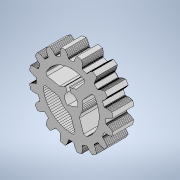
# Autodesk Inventor part: Ведущая шестерня дифференециала
Saved by Autodesk Inventor 2020 (Build 240168000, 168)
## iProperties
Created: 2021-05-23
Part Number: Ведущая шестерня дифференециала
Material: Типовые
Document SubType Name: Modeling
Designer: Антон
Density: 1 g/cm^3
Appearance: По умолчанию
Author: Антон
Autodesk Inventor part; units mm, degrees
note: some values were not read from the file. Chosen so that the rebuilt part matches the saved one: arc direction of "Выдавливание3".
(part 1 of 2)
ref_plane "YZ Plane" through (0, 0, 0) normal (1, 0, 0) x (0, 1, 0)
ref_plane "XZ Plane" through (0, 0, 0) normal (0, 1, 0) x (-1, 0, 0)
ref_plane "XY Plane" through (0, 0, 0) normal (0, 0, 1) x (1, 0, 0)
sketch "Эскиз1" plane through (0, 0, 0) normal (0, 0, 1) x (1, 0, 0)
  line L0 (0.5652, 9.3598) -> (0.528, 9.4555)
  line L1 (0.528, 9.4555) -> (0.4873, 9.4932)
  line L2 (0.4873, 9.4932) -> (0.446, 9.5204)
  line L3 (0.446, 9.5204) -> (0.3622, 9.5591)
  line L4 (0.3622, 9.5591) -> (0.2775, 9.5854)
  line L5 (0.2775, 9.5854) -> (0.1922, 9.604)
  line L6 (0.1922, 9.604) -> (0.0227, 9.6523)
  line L7 (0.0227, 9.6523) -> (-0.1453, 9.7165)
  line L8 (-0.1453, 9.7165) -> (-0.3118, 9.7933)
  line L9 (-0.3118, 9.7933) -> (-0.4767, 9.881)
  line L10 (-0.4767, 9.881) -> (-0.6399, 9.9788)
  line L11 (-0.6399, 9.9788) -> (-0.8013, 10.0859)
  line L12 (-0.8013, 10.0859) -> (-0.9608, 10.202)
  line L13 (-0.9608, 10.202) -> (-1.0789, 10.2947)
  line L14 (-1.0789, 10.2947) -> (-0.8657, 11.3669)
  line L15 (-0.8657, 11.3669) -> (-0.721, 11.4073)
  line L16 (-0.721, 11.4073) -> (-0.5293, 11.4535)
  line L17 (-0.5293, 11.4535) -> (-0.3392, 11.4907)
  line L18 (-0.3392, 11.4907) -> (-0.151, 11.5186)
  line L19 (-0.151, 11.5186) -> (0.035, 11.5365)
  line L20 (0.035, 11.5365) -> (0.2181, 11.5437)
  line L21 (0.2181, 11.5437) -> (0.3979, 11.5388)
  line L22 (0.3979, 11.5388) -> (0.573, 11.5185)
  line L23 (0.573, 11.5185) -> (0.659, 11.5031)
  line L24 (0.659, 11.5031) -> (0.7473, 11.4949)
  line L25 (0.7473, 11.4949) -> (0.8395, 11.4986)
  line L26 (0.8395, 11.4986) -> (0.8881, 11.5079)
  line L27 (0.8881, 11.5079) -> (0.9401, 11.5272)
  line L28 (0.9401, 11.5272) -> (1.0111, 11.6014)
  line L29 (1.0111, 11.6014) -> (1.3841, 12.5018)
  line L30 (1.3841, 12.5018) -> (1.3863, 12.6044)
  line L31 (1.3863, 12.6044) -> (1.3631, 12.6548)
  line L32 (1.3631, 12.6548) -> (1.3354, 12.6958)
  line L33 (1.3354, 12.6958) -> (1.2728, 12.7636)
  line L34 (1.2728, 12.7636) -> (1.2046, 12.8203)
  line L35 (1.2046, 12.8203) -> (1.1329, 12.8702)
  line L36 (1.1329, 12.8702) -> (0.9947, 12.9796)
  line L37 (0.9947, 12.9796) -> (0.8641, 13.1032)
  line L38 (0.8641, 13.1032) -> (0.7397, 13.2378)
  line L39 (0.7397, 13.2378) -> (0.6209, 13.382)
  line L40 (0.6209, 13.382) -> (0.5075, 13.5348)
  line L41 (0.5075, 13.5348) -> (0.3994, 13.6956)
  line L42 (0.3994, 13.6956) -> (0.2965, 13.8638)
  line L43 (0.2965, 13.8638) -> (0.2228, 13.9947)
  line L44 (0.2228, 13.9947) -> (0.8302, 14.9036)
  line L45 (0.8302, 14.9036) -> (0.9793, 14.8856)
  line L46 (0.9793, 14.8856) -> (1.1741, 14.8549)
  line L47 (1.1741, 14.8549) -> (1.364, 14.8166)
  line L48 (1.364, 14.8166) -> (1.5485, 14.7703)
  line L49 (1.5485, 14.7703) -> (1.7272, 14.7157)
  line L50 (1.7272, 14.7157) -> (1.8991, 14.6523)
  line L51 (1.8991, 14.6523) -> (2.0633, 14.5789)
  line L52 (2.0633, 14.5789) -> (2.2174, 14.4931)
  line L53 (2.2174, 14.4931) -> (2.2909, 14.446)
  line L54 (2.2909, 14.446) -> (2.3693, 14.4047)
  line L55 (2.3693, 14.4047) -> (2.4559, 14.3728)
  line L56 (2.4559, 14.3728) -> (2.5044, 14.3628)
  line L57 (2.5044, 14.3628) -> (2.5599, 14.3607)
  line L58 (2.5599, 14.3607) -> (2.6538, 14.4021)
  line L59 (2.6538, 14.4021) -> (3.3429, 15.0912)
  line L60 (3.3429, 15.0912) -> (3.3843, 15.1852)
  line L61 (3.3843, 15.1852) -> (3.3822, 15.2406)
  line L62 (3.3822, 15.2406) -> (3.3722, 15.2891)
  line L63 (3.3722, 15.2891) -> (3.3403, 15.3757)
  line L64 (3.3403, 15.3757) -> (3.299, 15.4541)
  line L65 (3.299, 15.4541) -> (3.2519, 15.5277)
  line L66 (3.2519, 15.5277) -> (3.1661, 15.6817)
  line L67 (3.1661, 15.6817) -> (3.0927, 15.8459)
  line L68 (3.0927, 15.8459) -> (3.0293, 16.0179)
  line L69 (3.0293, 16.0179) -> (2.9747, 16.1965)
  line L70 (2.9747, 16.1965) -> (2.9285, 16.381)
  line L71 (2.9285, 16.381) -> (2.8901, 16.5709)
  line L72 (2.8901, 16.5709) -> (2.8594, 16.7658)
  line L73 (2.8594, 16.7658) -> (2.8414, 16.9149)
  line L74 (2.8414, 16.9149) -> (3.7504, 17.5222)
  line L75 (3.7504, 17.5222) -> (3.8812, 17.4485)
  line L76 (3.8812, 17.4485) -> (4.0495, 17.3456)
  line L77 (4.0495, 17.3456) -> (4.2102, 17.2375)
  line L78 (4.2102, 17.2375) -> (4.363, 17.1241)
  line L79 (4.363, 17.1241) -> (4.5072, 17.0053)
  line L80 (4.5072, 17.0053) -> (4.6418, 16.8809)
  line L81 (4.6418, 16.8809) -> (4.7654, 16.7503)
  line L82 (4.7654, 16.7503) -> (4.8749, 16.6121)
  line L83 (4.8749, 16.6121) -> (4.9247, 16.5404)
  line L84 (4.9247, 16.5404) -> (4.9814, 16.4722)
  line L85 (4.9814, 16.4722) -> (5.0493, 16.4097)
  line L86 (5.0493, 16.4097) -> (5.0902, 16.3819)
  line L87 (5.0902, 16.3819) -> (5.1406, 16.3587)
  line L88 (5.1406, 16.3587) -> (5.2433, 16.3609)
  line L89 (5.2433, 16.3609) -> (6.1437, 16.7339)
  line L90 (6.1437, 16.7339) -> (6.2178, 16.8049)
  line L91 (6.2178, 16.8049) -> (6.2371, 16.8569)
  line L92 (6.2371, 16.8569) -> (6.2464, 16.9055)
  line L93 (6.2464, 16.9055) -> (6.2501, 16.9977)
  line L94 (6.2501, 16.9977) -> (6.242, 17.086)
  line L95 (6.242, 17.086) -> (6.2266, 17.172)
  line L96 (6.2266, 17.172) -> (6.2063, 17.3471)
  line L97 (6.2063, 17.3471) -> (6.2013, 17.5269)
  line L98 (6.2013, 17.5269) -> (6.2085, 17.71)
  line L99 (6.2085, 17.71) -> (6.2264, 17.896)
  line L100 (6.2264, 17.896) -> (6.2543, 18.0842)
  line L101 (6.2543, 18.0842) -> (6.2915, 18.2743)
  line L102 (6.2915, 18.2743) -> (6.3378, 18.466)
  line L103 (6.3378, 18.466) -> (6.3782, 18.6107)
  line L104 (6.3782, 18.6107) -> (7.4504, 18.824)
  line L105 (7.4504, 18.824) -> (7.543, 18.7058)
  line L106 (7.543, 18.7058) -> (7.6591, 18.5463)
  line L107 (7.6591, 18.5463) -> (7.7662, 18.3849)
  line L108 (7.7662, 18.3849) -> (7.864, 18.2217)
  line L109 (7.864, 18.2217) -> (7.9518, 18.0568)
  line L110 (7.9518, 18.0568) -> (8.0285, 17.8903)
  line L111 (8.0285, 17.8903) -> (8.0927, 17.7224)
  line L112 (8.0927, 17.7224) -> (8.141, 17.5528)
  line L113 (8.141, 17.5528) -> (8.1596, 17.4675)
  line L114 (8.1596, 17.4675) -> (8.1859, 17.3828)
  line L115 (8.1859, 17.3828) -> (8.2246, 17.299)
  line L116 (8.2246, 17.299) -> (8.2518, 17.2577)
  line L117 (8.2518, 17.2577) -> (8.2895, 17.217)
  line L118 (8.2895, 17.217) -> (8.3852, 17.1798)
  line L119 (8.3852, 17.1798) -> (9.3598, 17.1798)
  line L120 (9.3598, 17.1798) -> (9.4555, 17.217)
  line L121 (9.4555, 17.217) -> (9.4932, 17.2577)
  line L122 (9.4932, 17.2577) -> (9.5204, 17.299)
  line L123 (9.5204, 17.299) -> (9.5591, 17.3828)
  line L124 (9.5591, 17.3828) -> (9.5854, 17.4675)
  line L125 (9.5854, 17.4675) -> (9.604, 17.5528)
  line L126 (9.604, 17.5528) -> (9.6523, 17.7224)
  line L127 (9.6523, 17.7224) -> (9.7165, 17.8903)
  line L128 (9.7165, 17.8903) -> (9.7933, 18.0568)
  line L129 (9.7933, 18.0568) -> (9.881, 18.2217)
  line L130 (9.881, 18.2217) -> (9.9788, 18.3849)
  line L131 (9.9788, 18.3849) -> (10.0859, 18.5463)
  line L132 (10.0859, 18.5463) -> (10.202, 18.7058)
  line L133 (10.202, 18.7058) -> (10.2947, 18.824)
  line L134 (10.2947, 18.824) -> (11.3669, 18.6107)
  line L135 (11.3669, 18.6107) -> (11.4073, 18.466)
  line L136 (11.4073, 18.466) -> (11.4535, 18.2743)
  line L137 (11.4535, 18.2743) -> (11.4907, 18.0842)
  line L138 (11.4907, 18.0842) -> (11.5186, 17.896)
  line L139 (11.5186, 17.896) -> (11.5365, 17.71)
  line L140 (11.5365, 17.71) -> (11.5437, 17.5269)
  line L141 (11.5437, 17.5269) -> (11.5388, 17.3471)
  line L142 (11.5388, 17.3471) -> (11.5185, 17.172)
  line L143 (11.5185, 17.172) -> (11.5031, 17.086)
  line L144 (11.5031, 17.086) -> (11.4949, 16.9977)
  line L145 (11.4949, 16.9977) -> (11.4986, 16.9055)
  line L146 (11.4986, 16.9055) -> (11.5079, 16.8569)
  line L147 (11.5079, 16.8569) -> (11.5272, 16.8049)
  line L148 (11.5272, 16.8049) -> (11.6014, 16.7339)
  line L149 (11.6014, 16.7339) -> (12.5018, 16.3609)
  line L150 (12.5018, 16.3609) -> (12.6044, 16.3587)
  line L151 (12.6044, 16.3587) -> (12.6548, 16.3819)
  line L152 (12.6548, 16.3819) -> (12.6958, 16.4097)
  line L153 (12.6958, 16.4097) -> (12.7636, 16.4722)
  line L154 (12.7636, 16.4722) -> (12.8203, 16.5404)
  line L155 (12.8203, 16.5404) -> (12.8702, 16.6121)
  line L156 (12.8702, 16.6121) -> (12.9796, 16.7503)
  line L157 (12.9796, 16.7503) -> (13.1032, 16.8809)
  line L158 (13.1032, 16.8809) -> (13.2378, 17.0053)
  line L159 (13.2378, 17.0053) -> (13.382, 17.1241)
  line L160 (13.382, 17.1241) -> (13.5348, 17.2375)
  line L161 (13.5348, 17.2375) -> (13.6956, 17.3456)
  line L162 (13.6956, 17.3456) -> (13.8638, 17.4485)
  line L163 (13.8638, 17.4485) -> (13.9947, 17.5222)
  line L164 (13.9947, 17.5222) -> (14.9036, 16.9149)
  line L165 (14.9036, 16.9149) -> (14.8856, 16.7658)
  line L166 (14.8856, 16.7658) -> (14.8549, 16.5709)
  line L167 (14.8549, 16.5709) -> (14.8166, 16.381)
  line L168 (14.8166, 16.381) -> (14.7703, 16.1965)
  line L169 (14.7703, 16.1965) -> (14.7157, 16.0179)
  line L170 (14.7157, 16.0179) -> (14.6523, 15.8459)
  line L171 (14.6523, 15.8459) -> (14.5789, 15.6817)
  line L172 (14.5789, 15.6817) -> (14.4931, 15.5277)
  line L173 (14.4931, 15.5277) -> (14.446, 15.4541)
  line L174 (14.446, 15.4541) -> (14.4047, 15.3757)
  line L175 (14.4047, 15.3757) -> (14.3728, 15.2891)
  line L176 (14.3728, 15.2891) -> (14.3628, 15.2406)
  line L177 (14.3628, 15.2406) -> (14.3607, 15.1852)
  line L178 (14.3607, 15.1852) -> (14.4021, 15.0912)
  line L179 (14.4021, 15.0912) -> (15.0912, 14.4021)
  line L180 (15.0912, 14.4021) -> (15.1852, 14.3607)
  line L181 (15.1852, 14.3607) -> (15.2406, 14.3628)
  line L182 (15.2406, 14.3628) -> (15.2891, 14.3728)
  line L183 (15.2891, 14.3728) -> (15.3757, 14.4047)
  line L184 (15.3757, 14.4047) -> (15.4541, 14.446)
  line L185 (15.4541, 14.446) -> (15.5277, 14.4931)
  line L186 (15.5277, 14.4931) -> (15.6817, 14.5789)
  line L187 (15.6817, 14.5789) -> (15.8459, 14.6523)
  line L188 (15.8459, 14.6523) -> (16.0179, 14.7157)
  line L189 (16.0179, 14.7157) -> (16.1965, 14.7703)
  line L190 (16.1965, 14.7703) -> (16.381, 14.8166)
  line L191 (16.381, 14.8166) -> (16.5709, 14.8549)
  line L192 (16.5709, 14.8549) -> (16.7658, 14.8856)
  line L193 (16.7658, 14.8856) -> (16.9149, 14.9036)
  line L194 (16.9149, 14.9036) -> (17.5222, 13.9947)
  line L195 (17.5222, 13.9947) -> (17.4485, 13.8638)
  line L196 (17.4485, 13.8638) -> (17.3456, 13.6956)
  line L197 (17.3456, 13.6956) -> (17.2375, 13.5348)
  line L198 (17.2375, 13.5348) -> (17.1241, 13.382)
  line L199 (17.1241, 13.382) -> (17.0053, 13.2378)
  line L200 (17.0053, 13.2378) -> (16.8809, 13.1032)
  line L201 (16.8809, 13.1032) -> (16.7503, 12.9796)
  line L202 (16.7503, 12.9796) -> (16.6121, 12.8702)
  line L203 (16.6121, 12.8702) -> (16.5404, 12.8203)
  line L204 (16.5404, 12.8203) -> (16.4722, 12.7636)
  line L205 (16.4722, 12.7636) -> (16.4097, 12.6958)
  line L206 (16.4097, 12.6958) -> (16.3819, 12.6548)
  line L207 (16.3819, 12.6548) -> (16.3587, 12.6044)
  line L208 (16.3587, 12.6044) -> (16.3609, 12.5018)
  line L209 (16.3609, 12.5018) -> (16.7339, 11.6014)
  line L210 (16.7339, 11.6014) -> (16.8049, 11.5272)
  line L211 (16.8049, 11.5272) -> (16.8569, 11.5079)
  line L212 (16.8569, 11.5079) -> (16.9055, 11.4986)
  line L213 (16.9055, 11.4986) -> (16.9977, 11.4949)
  line L214 (16.9977, 11.4949) -> (17.086, 11.5031)
  line L215 (17.086, 11.5031) -> (17.172, 11.5185)
  line L216 (17.172, 11.5185) -> (17.3471, 11.5388)
  line L217 (17.3471, 11.5388) -> (17.5269, 11.5437)
  line L218 (17.5269, 11.5437) -> (17.71, 11.5365)
  line L219 (17.71, 11.5365) -> (17.896, 11.5186)
  line L220 (17.896, 11.5186) -> (18.0842, 11.4907)
  line L221 (18.0842, 11.4907) -> (18.2743, 11.4535)
  line L222 (18.2743, 11.4535) -> (18.466, 11.4073)
  line L223 (18.466, 11.4073) -> (18.6107, 11.3669)
  line L224 (18.6107, 11.3669) -> (18.824, 10.2947)
  line L225 (18.824, 10.2947) -> (18.7058, 10.202)
  line L226 (18.7058, 10.202) -> (18.5463, 10.0859)
  line L227 (18.5463, 10.0859) -> (18.3849, 9.9788)
  line L228 (18.3849, 9.9788) -> (18.2217, 9.881)
  line L229 (18.2217, 9.881) -> (18.0568, 9.7933)
  line L230 (18.0568, 9.7933) -> (17.8903, 9.7165)
  line L231 (17.8903, 9.7165) -> (17.7224, 9.6523)
  line L232 (17.7224, 9.6523) -> (17.5528, 9.604)
  line L233 (17.5528, 9.604) -> (17.4675, 9.5854)
  line L234 (17.4675, 9.5854) -> (17.3828, 9.5591)
  line L235 (17.3828, 9.5591) -> (17.299, 9.5204)
  line L236 (17.299, 9.5204) -> (17.2577, 9.4932)
  line L237 (17.2577, 9.4932) -> (17.217, 9.4555)
  line L238 (17.217, 9.4555) -> (17.1798, 9.3598)
  line L239 (17.1798, 9.3598) -> (17.1798, 8.3852)
  line L240 (17.1798, 8.3852) -> (17.217, 8.2895)
  line L241 (17.217, 8.2895) -> (17.2577, 8.2518)
  line L242 (17.2577, 8.2518) -> (17.299, 8.2246)
  line L243 (17.299, 8.2246) -> (17.3828, 8.1859)
  line L244 (17.3828, 8.1859) -> (17.4675, 8.1596)
  line L245 (17.4675, 8.1596) -> (17.5528, 8.141)
  line L246 (17.5528, 8.141) -> (17.7224, 8.0927)
  line L247 (17.7224, 8.0927) -> (17.8903, 8.0285)
  line L248 (17.8903, 8.0285) -> (18.0568, 7.9518)
  line L249 (18.0568, 7.9518) -> (18.2217, 7.864)
  line L250 (18.2217, 7.864) -> (18.3849, 7.7662)
  line L251 (18.3849, 7.7662) -> (18.5463, 7.6591)
  line L252 (18.5463, 7.6591) -> (18.7058, 7.543)
  line L253 (18.7058, 7.543) -> (18.824, 7.4504)
  line L254 (18.824, 7.4504) -> (18.6107, 6.3782)
  line L255 (18.6107, 6.3782) -> (18.466, 6.3378)
  line L256 (18.466, 6.3378) -> (18.2743, 6.2915)
  line L257 (18.2743, 6.2915) -> (18.0842, 6.2543)
  line L258 (18.0842, 6.2543) -> (17.896, 6.2264)
  line L259 (17.896, 6.2264) -> (17.71, 6.2085)
  line L260 (17.71, 6.2085) -> (17.5269, 6.2013)
  line L261 (17.5269, 6.2013) -> (17.3471, 6.2063)
  line L262 (17.3471, 6.2063) -> (17.172, 6.2266)
  line L263 (17.172, 6.2266) -> (17.086, 6.242)
  line L264 (17.086, 6.242) -> (16.9977, 6.2501)
  line L265 (16.9977, 6.2501) -> (16.9055, 6.2464)
  line L266 (16.9055, 6.2464) -> (16.8569, 6.2371)
  line L267 (16.8569, 6.2371) -> (16.8049, 6.2178)
  line L268 (16.8049, 6.2178) -> (16.7339, 6.1437)
  line L269 (16.7339, 6.1437) -> (16.3609, 5.2433)
  line L270 (16.3609, 5.2433) -> (16.3587, 5.1406)
  line L271 (16.3587, 5.1406) -> (16.3819, 5.0902)
  line L272 (16.3819, 5.0902) -> (16.4097, 5.0493)
  line L273 (16.4097, 5.0493) -> (16.4722, 4.9814)
  line L274 (16.4722, 4.9814) -> (16.5404, 4.9247)
  line L275 (16.5404, 4.9247) -> (16.6121, 4.8749)
  line L276 (16.6121, 4.8749) -> (16.7503, 4.7654)
  line L277 (16.7503, 4.7654) -> (16.8809, 4.6418)
  line L278 (16.8809, 4.6418) -> (17.0053, 4.5072)
  line L279 (17.0053, 4.5072) -> (17.1241, 4.363)
  line L280 (17.1241, 4.363) -> (17.2375, 4.2102)
  line L281 (17.2375, 4.2102) -> (17.3456, 4.0495)
  line L282 (17.3456, 4.0495) -> (17.4485, 3.8812)
  line L283 (17.4485, 3.8812) -> (17.5222, 3.7504)
  line L284 (17.5222, 3.7504) -> (16.9149, 2.8414)
  line L285 (16.9149, 2.8414) -> (16.7658, 2.8594)
  line L286 (16.7658, 2.8594) -> (16.5709, 2.8901)
  line L287 (16.5709, 2.8901) -> (16.381, 2.9285)
  line L288 (16.381, 2.9285) -> (16.1965, 2.9747)
  line L289 (16.1965, 2.9747) -> (16.0179, 3.0293)
  line L290 (16.0179, 3.0293) -> (15.8459, 3.0927)
  line L291 (15.8459, 3.0927) -> (15.6817, 3.1661)
  line L292 (15.6817, 3.1661) -> (15.5277, 3.2519)
  line L293 (15.5277, 3.2519) -> (15.4541, 3.299)
  line L294 (15.4541, 3.299) -> (15.3757, 3.3403)
  line L295 (15.3757, 3.3403) -> (15.2891, 3.3722)
  line L296 (15.2891, 3.3722) -> (15.2406, 3.3822)
  line L297 (15.2406, 3.3822) -> (15.1852, 3.3843)
  line L298 (15.1852, 3.3843) -> (15.0912, 3.3429)
  line L299 (15.0912, 3.3429) -> (14.4021, 2.6538)
  line L300 (14.4021, 2.6538) -> (14.3607, 2.5599)
  line L301 (14.3607, 2.5599) -> (14.3628, 2.5044)
  line L302 (14.3628, 2.5044) -> (14.3728, 2.4559)
  line L303 (14.3728, 2.4559) -> (14.4047, 2.3693)
  line L304 (14.4047, 2.3693) -> (14.446, 2.2909)
  line L305 (14.446, 2.2909) -> (14.4931, 2.2174)
  line L306 (14.4931, 2.2174) -> (14.5789, 2.0633)
  line L307 (14.5789, 2.0633) -> (14.6523, 1.8991)
  line L308 (14.6523, 1.8991) -> (14.7157, 1.7272)
  line L309 (14.7157, 1.7272) -> (14.7703, 1.5485)
  line L310 (14.7703, 1.5485) -> (14.8166, 1.364)
  line L311 (14.8166, 1.364) -> (14.8549, 1.1741)
  line L312 (14.8549, 1.1741) -> (14.8856, 0.9793)
  line L313 (14.8856, 0.9793) -> (14.9036, 0.8302)
  line L314 (14.9036, 0.8302) -> (13.9947, 0.2228)
  line L315 (13.9947, 0.2228) -> (13.8638, 0.2965)
  line L316 (13.8638, 0.2965) -> (13.6956, 0.3994)
  line L317 (13.6956, 0.3994) -> (13.5348, 0.5075)
  line L318 (13.5348, 0.5075) -> (13.382, 0.6209)
  line L319 (13.382, 0.6209) -> (13.2378, 0.7397)
  line L320 (13.2378, 0.7397) -> (13.1032, 0.8641)
  line L321 (13.1032, 0.8641) -> (12.9796, 0.9947)
  line L322 (12.9796, 0.9947) -> (12.8702, 1.1329)
  line L323 (12.8702, 1.1329) -> (12.8203, 1.2046)
  line L324 (12.8203, 1.2046) -> (12.7636, 1.2728)
  line L325 (12.7636, 1.2728) -> (12.6958, 1.3354)
  line L326 (12.6958, 1.3354) -> (12.6548, 1.3631)
  line L327 (12.6548, 1.3631) -> (12.6044, 1.3863)
  line L328 (12.6044, 1.3863) -> (12.5018, 1.3841)
  line L329 (12.5018, 1.3841) -> (11.6014, 1.0111)
  line L330 (11.6014, 1.0111) -> (11.5272, 0.9401)
  line L331 (11.5272, 0.9401) -> (11.5079, 0.8881)
  line L332 (11.5079, 0.8881) -> (11.4986, 0.8395)
  line L333 (11.4986, 0.8395) -> (11.4949, 0.7473)
  line L334 (11.4949, 0.7473) -> (11.5031, 0.659)
  line L335 (11.5031, 0.659) -> (11.5185, 0.573)
  line L336 (11.5185, 0.573) -> (11.5388, 0.3979)
  line L337 (11.5388, 0.3979) -> (11.5437, 0.2181)
  line L338 (11.5437, 0.2181) -> (11.5365, 0.035)
  line L339 (11.5365, 0.035) -> (11.5186, -0.151)
  line L340 (11.5186, -0.151) -> (11.4907, -0.3392)
  line L341 (11.4907, -0.3392) -> (11.4535, -0.5293)
  line L342 (11.4535, -0.5293) -> (11.4073, -0.721)
  line L343 (11.4073, -0.721) -> (11.3669, -0.8657)
  line L344 (11.3669, -0.8657) -> (10.2947, -1.0789)
  line L345 (10.2947, -1.0789) -> (10.202, -0.9608)
  line L346 (10.202, -0.9608) -> (10.0859, -0.8013)
  line L347 (10.0859, -0.8013) -> (9.9788, -0.6399)
  line L348 (9.9788, -0.6399) -> (9.881, -0.4767)
  line L349 (9.881, -0.4767) -> (9.7933, -0.3118)
  line L350 (9.7933, -0.3118) -> (9.7165, -0.1453)
  line L351 (9.7165, -0.1453) -> (9.6523, 0.0227)
  line L352 (9.6523, 0.0227) -> (9.604, 0.1922)
  line L353 (9.604, 0.1922) -> (9.5854, 0.2775)
  line L354 (9.5854, 0.2775) -> (9.5591, 0.3622)
  line L355 (9.5591, 0.3622) -> (9.5204, 0.446)
  line L356 (9.5204, 0.446) -> (9.4932, 0.4873)
  line L357 (9.4932, 0.4873) -> (9.4555, 0.528)
  line L358 (9.4555, 0.528) -> (9.3598, 0.5652)
  line L359 (9.3598, 0.5652) -> (8.3852, 0.5652)
  line L360 (8.3852, 0.5652) -> (8.2895, 0.528)
  line L361 (8.2895, 0.528) -> (8.2518, 0.4873)
  line L362 (8.2518, 0.4873) -> (8.2246, 0.446)
  line L363 (8.2246, 0.446) -> (8.1859, 0.3622)
  line L364 (8.1859, 0.3622) -> (8.1596, 0.2775)
  line L365 (8.1596, 0.2775) -> (8.141, 0.1922)
  line L366 (8.141, 0.1922) -> (8.0927, 0.0227)
  line L367 (8.0927, 0.0227) -> (8.0285, -0.1453)
  line L368 (8.0285, -0.1453) -> (7.9518, -0.3118)
  line L369 (7.9518, -0.3118) -> (7.864, -0.4767)
  line L370 (7.864, -0.4767) -> (7.7662, -0.6399)
  line L371 (7.7662, -0.6399) -> (7.6591, -0.8013)
  line L372 (7.6591, -0.8013) -> (7.543, -0.9608)
  line L373 (7.543, -0.9608) -> (7.4504, -1.0789)
  line L374 (7.4504, -1.0789) -> (6.3782, -0.8657)
  line L375 (6.3782, -0.8657) -> (6.3378, -0.721)
  line L376 (6.3378, -0.721) -> (6.2915, -0.5293)
  line L377 (6.2915, -0.5293) -> (6.2543, -0.3392)
  line L378 (6.2543, -0.3392) -> (6.2264, -0.151)
  line L379 (6.2264, -0.151) -> (6.2085, 0.035)
  line L380 (6.2085, 0.035) -> (6.2013, 0.2181)
  line L381 (6.2013, 0.2181) -> (6.2063, 0.3979)
  line L382 (6.2063, 0.3979) -> (6.2266, 0.573)
  line L383 (6.2266, 0.573) -> (6.242, 0.659)
  line L384 (6.242, 0.659) -> (6.2501, 0.7473)
  line L385 (6.2501, 0.7473) -> (6.2464, 0.8395)
  line L386 (6.2464, 0.8395) -> (6.2371, 0.8881)
  line L387 (6.2371, 0.8881) -> (6.2178, 0.9401)
  line L388 (6.2178, 0.9401) -> (6.1437, 1.0111)
  line L389 (6.1437, 1.0111) -> (5.2433, 1.3841)
  line L390 (5.2433, 1.3841) -> (5.1406, 1.3863)
  line L391 (5.1406, 1.3863) -> (5.0902, 1.3631)
  line L392 (5.0902, 1.3631) -> (5.0493, 1.3354)
  line L393 (5.0493, 1.3354) -> (4.9814, 1.2728)
  line L394 (4.9814, 1.2728) -> (4.9247, 1.2046)
  line L395 (4.9247, 1.2046) -> (4.8749, 1.1329)
  line L396 (4.8749, 1.1329) -> (4.7654, 0.9947)
  line L397 (4.7654, 0.9947) -> (4.6418, 0.8641)
  line L398 (4.6418, 0.8641) -> (4.5072, 0.7397)
  line L399 (4.5072, 0.7397) -> (4.363, 0.6209)
  line L400 (4.363, 0.6209) -> (4.2102, 0.5075)
  line L401 (4.2102, 0.5075) -> (4.0495, 0.3994)
  line L402 (4.0495, 0.3994) -> (3.8812, 0.2965)
  line L403 (3.8812, 0.2965) -> (3.7504, 0.2228)
  line L404 (3.7504, 0.2228) -> (2.8414, 0.8302)
  line L405 (2.8414, 0.8302) -> (2.8594, 0.9793)
  line L406 (2.8594, 0.9793) -> (2.8901, 1.1741)
  line L407 (2.8901, 1.1741) -> (2.9285, 1.364)
  line L408 (2.9285, 1.364) -> (2.9747, 1.5485)
  line L409 (2.9747, 1.5485) -> (3.0293, 1.7272)
  line L410 (3.0293, 1.7272) -> (3.0927, 1.8991)
  line L411 (3.0927, 1.8991) -> (3.1661, 2.0633)
  line L412 (3.1661, 2.0633) -> (3.2519, 2.2174)
  line L413 (3.2519, 2.2174) -> (3.299, 2.2909)
  line L414 (3.299, 2.2909) -> (3.3403, 2.3693)
  line L415 (3.3403, 2.3693) -> (3.3722, 2.4559)
  line L416 (3.3722, 2.4559) -> (3.3822, 2.5044)
  line L417 (3.3822, 2.5044) -> (3.3843, 2.5599)
  line L418 (3.3843, 2.5599) -> (3.3429, 2.6538)
  line L419 (3.3429, 2.6538) -> (2.6538, 3.3429)
  line L420 (2.6538, 3.3429) -> (2.5599, 3.3843)
  line L421 (2.5599, 3.3843) -> (2.5044, 3.3822)
  line L422 (2.5044, 3.3822) -> (2.4559, 3.3722)
  line L423 (2.4559, 3.3722) -> (2.3693, 3.3403)
  line L424 (2.3693, 3.3403) -> (2.2909, 3.299)
  line L425 (2.2909, 3.299) -> (2.2174, 3.2519)
  line L426 (2.2174, 3.2519) -> (2.0633, 3.1661)
  line L427 (2.0633, 3.1661) -> (1.8991, 3.0927)
  line L428 (1.8991, 3.0927) -> (1.7272, 3.0293)
  line L429 (1.7272, 3.0293) -> (1.5485, 2.9747)
  line L430 (1.5485, 2.9747) -> (1.364, 2.9285)
  line L431 (1.364, 2.9285) -> (1.1741, 2.8901)
  line L432 (1.1741, 2.8901) -> (0.9793, 2.8594)
  line L433 (0.9793, 2.8594) -> (0.8302, 2.8414)
  line L434 (0.8302, 2.8414) -> (0.2228, 3.7504)
  line L435 (0.2228, 3.7504) -> (0.2965, 3.8812)
  line L436 (0.2965, 3.8812) -> (0.3994, 4.0495)
  line L437 (0.3994, 4.0495) -> (0.5075, 4.2102)
  line L438 (0.5075, 4.2102) -> (0.6209, 4.363)
  line L439 (0.6209, 4.363) -> (0.7397, 4.5072)
  line L440 (0.7397, 4.5072) -> (0.8641, 4.6418)
  line L441 (0.8641, 4.6418) -> (0.9947, 4.7654)
  line L442 (0.9947, 4.7654) -> (1.1329, 4.8749)
  line L443 (1.1329, 4.8749) -> (1.2046, 4.9247)
  line L444 (1.2046, 4.9247) -> (1.2728, 4.9814)
  line L445 (1.2728, 4.9814) -> (1.3354, 5.0493)
  line L446 (1.3354, 5.0493) -> (1.3631, 5.0902)
  line L447 (1.3631, 5.0902) -> (1.3863, 5.1406)
  line L448 (1.3863, 5.1406) -> (1.3841, 5.2433)
  line L449 (1.3841, 5.2433) -> (1.0111, 6.1437)
  line L450 (1.0111, 6.1437) -> (0.9401, 6.2178)
  line L451 (0.9401, 6.2178) -> (0.8881, 6.2371)
  line L452 (0.8881, 6.2371) -> (0.8395, 6.2464)
  line L453 (0.8395, 6.2464) -> (0.7473, 6.2501)
  line L454 (0.7473, 6.2501) -> (0.659, 6.242)
  line L455 (0.659, 6.242) -> (0.573, 6.2266)
  line L456 (0.573, 6.2266) -> (0.3979, 6.2063)
  line L457 (0.3979, 6.2063) -> (0.2181, 6.2013)
  line L458 (0.2181, 6.2013) -> (0.035, 6.2085)
  line L459 (0.035, 6.2085) -> (-0.151, 6.2264)
  line L460 (-0.151, 6.2264) -> (-0.3392, 6.2543)
  line L461 (-0.3392, 6.2543) -> (-0.5293, 6.2915)
  line L462 (-0.5293, 6.2915) -> (-0.721, 6.3378)
  line L463 (-0.721, 6.3378) -> (-0.8657, 6.3782)
  line L464 (-0.8657, 6.3782) -> (-1.0789, 7.4504)
  line L465 (-1.0789, 7.4504) -> (-0.9608, 7.543)
  line L466 (-0.9608, 7.543) -> (-0.8013, 7.6591)
  line L467 (-0.8013, 7.6591) -> (-0.6399, 7.7662)
  line L468 (-0.6399, 7.7662) -> (-0.4767, 7.864)
  line L469 (-0.4767, 7.864) -> (-0.3118, 7.9518)
  line L470 (-0.3118, 7.9518) -> (-0.1453, 8.0285)
  line L471 (-0.1453, 8.0285) -> (0.0227, 8.0927)
  line L472 (0.0227, 8.0927) -> (0.1922, 8.141)
  line L473 (0.1922, 8.141) -> (0.2775, 8.1596)
  line L474 (0.2775, 8.1596) -> (0.3622, 8.1859)
  line L475 (0.3622, 8.1859) -> (0.446, 8.2246)
  line L476 (0.446, 8.2246) -> (0.4873, 8.2518)
  line L477 (0.4873, 8.2518) -> (0.528, 8.2895)
  line L478 (0.528, 8.2895) -> (0.5652, 8.3852)
  line L479 (0.5652, 8.3852) -> (0.5652, 9.3598)
  line L480 (5.6712, 8.4057) -> (2.7091, 8.995)
  line L481 (2.7091, 8.995) -> (2.1823, 8.548)
  line L482 (2.1823, 8.548) -> (2.2189, 8.1017)
  line L483 (2.2189, 8.1017) -> (2.2853, 7.6589)
  line L484 (2.2853, 7.6589) -> (2.3811, 7.2214)
  line L485 (2.3811, 7.2214) -> (2.5059, 6.7914)
  line L486 (2.5059, 6.7914) -> (2.6592, 6.3707)
  line L487 (2.6592, 6.3707) -> (2.8403, 5.9611)
  line L488 (2.8403, 5.9611) -> (3.0483, 5.5646)
  line L489 (3.0483, 5.5646) -> (3.2823, 5.1828)
  line L490 (3.2823, 5.1828) -> (3.5413, 4.8176)
  line L491 (3.5413, 4.8176) -> (3.8242, 4.4704)
  line L492 (3.8242, 4.4704) -> (4.1296, 4.143)
  line L493 (4.1296, 4.143) -> (4.4562, 3.8366)
  line L494 (4.4562, 3.8366) -> (4.8025, 3.5528)
  line L495 (4.8025, 3.5528) -> (5.167, 3.2928)
  line L496 (5.167, 3.2928) -> (5.5481, 3.0576)
  line L497 (5.5481, 3.0576) -> (5.9441, 2.8485)
  line L498 (5.9441, 2.8485) -> (6.3531, 2.6663)
  line L499 (6.3531, 2.6663) -> (6.7734, 2.5119)
  line L500 (6.7734, 2.5119) -> (7.2031, 2.3858)
  line L501 (7.2031, 2.3858) -> (7.6402, 2.2888)
  line L502 (7.6402, 2.2888) -> (8.0829, 2.2211)
  line L503 (8.0829, 2.2211) -> (8.5291, 2.1833)
  line L504 (8.5291, 2.1833) -> (8.9768, 2.1752)
  line L505 (8.9768, 2.1752) -> (9.424, 2.1972)
  line L506 (9.424, 2.1972) -> (9.7984, 2.7778)
  line L507 (9.7984, 2.7778) -> (8.8276, 5.6377)
  line L508 (8.8276, 5.6377) -> (8.0411, 6.271)
  line L509 (8.0411, 6.271) -> (7.6939, 6.4087)
  line L510 (7.6939, 6.4087) -> (7.3688, 6.5926)
  line L511 (7.3688, 6.5926) -> (7.0717, 6.8191)
  line L512 (7.0717, 6.8191) -> (6.8084, 7.084)
  line L513 (6.8084, 7.084) -> (6.5837, 7.3824)
  line L514 (6.5837, 7.3824) -> (6.4017, 7.7087)
  line L515 (6.4017, 7.7087) -> (5.6712, 8.4057)
  line L516 (10.8774, 6.3335) -> (11.8482, 3.4736)
  line L517 (11.8482, 3.4736) -> (12.4987, 3.2409)
  line L518 (12.4987, 3.2409) -> (12.8668, 3.4958)
  line L519 (12.8668, 3.4958) -> (13.2172, 3.7746)
  line L520 (13.2172, 3.7746) -> (13.5481, 4.0763)
  line L521 (13.5481, 4.0763) -> (13.8581, 4.3994)
  line L522 (13.8581, 4.3994) -> (14.1458, 4.7425)
  line L523 (14.1458, 4.7425) -> (14.41, 5.1041)
  line L524 (14.41, 5.1041) -> (14.6494, 5.4825)
  line L525 (14.6494, 5.4825) -> (14.863, 5.8761)
  line L526 (14.863, 5.8761) -> (15.0498, 6.283)
  line L527 (15.0498, 6.283) -> (15.209, 6.7015)
  line L528 (15.209, 6.7015) -> (15.3399, 7.1298)
  line L529 (15.3399, 7.1298) -> (15.4419, 7.5658)
  line L530 (15.4419, 7.5658) -> (15.5145, 8.0076)
  line L531 (15.5145, 8.0076) -> (15.5574, 8.4533)
  line L532 (15.5574, 8.4533) -> (15.5705, 8.9009)
  line L533 (15.5705, 8.9009) -> (15.5537, 9.3484)
  line L534 (15.5537, 9.3484) -> (15.5069, 9.7937)
  line L535 (15.5069, 9.7937) -> (15.4305, 10.235)
  line L536 (15.4305, 10.235) -> (15.3249, 10.6701)
  line L537 (15.3249, 10.6701) -> (15.1903, 11.0972)
  line L538 (15.1903, 11.0972) -> (15.0276, 11.5143)
  line L539 (15.0276, 11.5143) -> (14.8373, 11.9197)
  line L540 (14.8373, 11.9197) -> (14.6204, 12.3114)
  line L541 (14.6204, 12.3114) -> (14.3778, 12.6878)
  line L542 (14.3778, 12.6878) -> (13.6877, 12.7217)
  line L543 (13.6877, 12.7217) -> (11.6964, 10.451)
  line L544 (11.6964, 10.451) -> (11.5412, 9.4533)
  line L545 (11.5412, 9.4533) -> (11.5955, 9.0837)
  line L546 (11.5955, 9.0837) -> (11.5988, 8.7102)
  line L547 (11.5988, 8.7102) -> (11.5512, 8.3397)
  line L548 (11.5512, 8.3397) -> (11.4534, 7.9792)
  line L549 (11.4534, 7.9792) -> (11.3074, 7.6353)
  line L550 (11.3074, 7.6353) -> (11.1158, 7.3147)
  line L551 (11.1158, 7.3147) -> (10.8774, 6.3335)
  line L552 (10.0689, 11.8783) -> (12.0603, 14.149)
  line L553 (12.0603, 14.149) -> (11.9366, 14.8287)
  line L554 (11.9366, 14.8287) -> (11.5318, 15.0201)
  line L555 (11.5318, 15.0201) -> (11.1151, 15.184)
  line L556 (11.1151, 15.184) -> (10.6883, 15.3197)
  line L557 (10.6883, 15.3197) -> (10.2535, 15.4267)
  line L558 (10.2535, 15.4267) -> (9.8125, 15.5043)
  line L559 (9.8125, 15.5043) -> (9.3673, 15.5523)
  line L560 (9.3673, 15.5523) -> (8.9199, 15.5704)
  line L561 (8.9199, 15.5704) -> (8.4723, 15.5586)
  line L562 (8.4723, 15.5586) -> (8.0264, 15.5169)
  line L563 (8.0264, 15.5169) -> (7.5844, 15.4455)
  line L564 (7.5844, 15.4455) -> (7.1481, 15.3448)
  line L565 (7.1481, 15.3448) -> (6.7195, 15.2151)
  line L566 (6.7195, 15.2151) -> (6.3005, 15.0571)
  line L567 (6.3005, 15.0571) -> (5.893, 14.8714)
  line L568 (5.893, 14.8714) -> (5.4989, 14.6589)
  line L569 (5.4989, 14.6589) -> (5.1198, 14.4206)
  line L570 (5.1198, 14.4206) -> (4.7575, 14.1575)
  line L571 (4.7575, 14.1575) -> (4.4136, 13.8707)
  line L572 (4.4136, 13.8707) -> (4.0896, 13.5616)
  line L573 (4.0896, 13.5616) -> (3.787, 13.2316)
  line L574 (3.787, 13.2316) -> (3.5071, 12.882)
  line L575 (3.5071, 12.882) -> (3.2512, 12.5146)
  line L576 (3.2512, 12.5146) -> (3.0204, 12.1308)
  line L577 (3.0204, 12.1308) -> (2.8158, 11.7326)
  line L578 (2.8158, 11.7326) -> (3.1314, 11.118)
  line L579 (3.1314, 11.118) -> (6.0935, 10.5288)
  line L580 (6.0935, 10.5288) -> (7.0352, 10.8933)
  line L581 (7.0352, 10.8933) -> (7.3281, 11.1251)
  line L582 (7.3281, 11.1251) -> (7.6499, 11.3147)
  line L583 (7.6499, 11.3147) -> (7.9946, 11.4587)
  line L584 (7.9946, 11.4587) -> (8.3557, 11.5543)
  line L585 (8.3557, 11.5543) -> (8.7265, 11.5998)
  line L586 (8.7265, 11.5998) -> (9.1, 11.5942)
  line L587 (9.1, 11.5942) -> (10.0689, 11.8783)
  circle A0 centre (8.8725, 8.8725) radius 0.5665
  line L588 (5.5217, 8.8725) -> (12.2234, 8.8725)
  line L589 (8.8725, 5.5217) -> (8.8725, 12.2234)
  point P0 (0, 0)
  constraints: 1180 end point, 1 centre point
extrude "Выдавливание1" add sketch "Эскиз1" along normal blind 5
sketch "Эскиз2" plane through (0, 0, 5) normal (0, 0, 1) x (1, 0, 0)
  circle A0 centre (8.8725, 8.8725) radius 0.5665 projected
  circle A1 centre (8.8725, 8.8725) radius 1.6
  line L0 (7.036, 9.3051) -> (7.6789, 7.4113)
  line L1 (7.6789, 7.4113) -> (10.709, 8.4399)
  line L2 (10.709, 8.4399) -> (10.0662, 10.3337)
  line L3 (10.0662, 10.3337) -> (7.036, 9.3051)
  line L4 (7.036, 9.3051) -> (10.709, 8.4399) construction
  line L5 (7.6789, 7.4113) -> (10.0662, 10.3337) construction
  line L6 (7.9946, 11.4587) -> (7.6499, 11.3147) projected
  line L7 (8.3557, 11.5543) -> (7.9946, 11.4587) projected
  line L8 (7.5211, 11.298) -> (8.4681, 11.6194)
  line L9 (8.4681, 11.6194) -> (9.0245, 9.9802)
  line L10 (9.0245, 9.9802) -> (8.0776, 9.6587)
  line L11 (8.0776, 9.6587) -> (7.5211, 11.298)
  point P0 (0, 0)
  point P1 (8.5511, 9.8194)
  point P2 (8.8574, 10.4724)
  point P3 (7.9105, 10.151)
  point P4 (8.0112, 7.5241)
  point P5 (10.3767, 8.3271)
  dimension "d2" = 3.2
  dimension "d3" = 2
  dimension "d6" = 1
  constraints: 20 end point, 5 midpoint, 4 parallel, 3 perpendicular, 1 centre point, 1 coincident, 1 tangent
  measures "d2" diameter of A1
  measures "d3" distance of L2.end L1.end
  measures "d6" distance of L9.end L10.end
extrude "Выдавливание2" cut sketch "Эскиз2" against normal through all contours A1 L1 L3 | L3 L9 A1 | L9 L3 L11 A1 | A1 L11 L8 L9 | L11 L3 A1
sketch "Эскиз3" plane through (0, 0, 0) normal (0, 0, -1) x (-1, 0, 0)
  line L0 (-8.8574, 10.4724) -> (-8.4848, 11.5701) projected
  line L1 (-8.7265, 11.5998) -> (-8.4848, 11.5701) projected
  line L2 (-9.1, 11.5942) -> (-8.7265, 11.5998) projected
  line L3 (-10.0689, 11.8783) -> (-9.1, 11.5942) projected
  line L4 (-12.0603, 14.149) -> (-10.0689, 11.8783) projected
  line L5 (-11.9366, 14.8287) -> (-12.0603, 14.149) projected
  line L6 (-11.5318, 15.0201) -> (-11.9366, 14.8287) projected
  line L7 (-11.1151, 15.184) -> (-11.5318, 15.0201) projected
  line L8 (-10.6883, 15.3197) -> (-11.1151, 15.184) projected
  line L9 (-10.2535, 15.4267) -> (-10.6883, 15.3197) projected
  line L10 (-9.8125, 15.5043) -> (-10.2535, 15.4267) projected
  line L11 (-9.3673, 15.5523) -> (-9.8125, 15.5043) projected
  line L12 (-8.9199, 15.5704) -> (-9.3673, 15.5523) projected
  line L13 (-8.4723, 15.5586) -> (-8.9199, 15.5704) projected
  line L14 (-8.0264, 15.5169) -> (-8.4723, 15.5586) projected
  line L15 (-7.5844, 15.4455) -> (-8.0264, 15.5169) projected
  line L16 (-7.1481, 15.3448) -> (-7.5844, 15.4455) projected
  line L17 (-6.7195, 15.2151) -> (-7.1481, 15.3448) projected
  line L18 (-6.3005, 15.0571) -> (-6.7195, 15.2151) projected
  line L19 (-5.893, 14.8714) -> (-6.3005, 15.0571) projected
  line L20 (-5.4989, 14.6589) -> (-5.893, 14.8714) projected
  line L21 (-5.1198, 14.4206) -> (-5.4989, 14.6589) projected
  line L22 (-4.7575, 14.1575) -> (-5.1198, 14.4206) projected
  line L23 (-4.4136, 13.8707) -> (-4.7575, 14.1575) projected
  line L24 (-4.0896, 13.5616) -> (-4.4136, 13.8707) projected
  line L25 (-3.787, 13.2316) -> (-4.0896, 13.5616) projected
  line L26 (-3.5071, 12.882) -> (-3.787, 13.2316) projected
  line L27 (-3.2512, 12.5146) -> (-3.5071, 12.882) projected
  line L28 (-3.0204, 12.1308) -> (-3.2512, 12.5146) projected
  line L29 (-2.8158, 11.7326) -> (-3.0204, 12.1308) projected
  line L30 (-3.1314, 11.118) -> (-2.8158, 11.7326) projected
  line L31 (-6.0935, 10.5288) -> (-3.1314, 11.118) projected
  line L32 (-7.0352, 10.8933) -> (-6.0935, 10.5288) projected
  line L33 (-7.3281, 11.1251) -> (-7.0352, 10.8933) projected
  line L34 (-7.5379, 11.2487) -> (-7.3281, 11.1251) projected
  line L35 (-7.5379, 11.2487) -> (-7.9105, 10.151) projected
  arc A0 (-8.0112, 7.5241) -> (-7.9105, 10.151) centre (-8.8725, 8.8725) ccw projected
  line L36 (-8.0112, 7.5241) -> (-10.3767, 8.3271) projected
  arc A1 (-8.8574, 10.4724) -> (-10.3767, 8.3271) centre (-8.8725, 8.8725) ccw projected
  line L37 (-11.5186, 17.896) -> (-11.4907, 18.0842) projected
  line L38 (-11.5365, 17.71) -> (-11.5186, 17.896) projected
  line L39 (-11.5437, 17.5269) -> (-11.5365, 17.71) projected
  line L40 (-11.5388, 17.3471) -> (-11.5437, 17.5269) projected
  line L41 (-11.5185, 17.172) -> (-11.5388, 17.3471) projected
  line L42 (-11.5031, 17.086) -> (-11.5185, 17.172) projected
  line L43 (-11.4949, 16.9977) -> (-11.5031, 17.086) projected
  line L44 (-11.4986, 16.9055) -> (-11.4949, 16.9977) projected
  line L45 (-11.5079, 16.8569) -> (-11.4986, 16.9055) projected
  line L46 (-11.5272, 16.8049) -> (-11.5079, 16.8569) projected
  line L47 (-11.6014, 16.7339) -> (-11.5272, 16.8049) projected
  line L48 (-12.5018, 16.3609) -> (-11.6014, 16.7339) projected
  line L49 (-12.6044, 16.3587) -> (-12.5018, 16.3609) projected
  line L50 (-12.6548, 16.3819) -> (-12.6044, 16.3587) projected
  line L51 (-12.6958, 16.4097) -> (-12.6548, 16.3819) projected
  line L52 (-12.7636, 16.4722) -> (-12.6958, 16.4097) projected
  line L53 (-12.8203, 16.5404) -> (-12.7636, 16.4722) projected
  line L54 (-12.8702, 16.6121) -> (-12.8203, 16.5404) projected
  line L55 (-12.9796, 16.7503) -> (-12.8702, 16.6121) projected
  line L56 (-13.1032, 16.8809) -> (-12.9796, 16.7503) projected
  line L57 (-13.2378, 17.0053) -> (-13.1032, 16.8809) projected
  line L58 (-13.382, 17.1241) -> (-13.2378, 17.0053) projected
  line L59 (-13.5348, 17.2375) -> (-13.382, 17.1241) projected
  line L60 (-13.6956, 17.3456) -> (-13.5348, 17.2375) projected
  line L61 (-13.8638, 17.4485) -> (-13.6956, 17.3456) projected
  line L62 (-13.9947, 17.5222) -> (-13.8638, 17.4485) projected
  line L63 (-14.9036, 16.9149) -> (-13.9947, 17.5222) projected
  line L64 (-14.8856, 16.7658) -> (-14.9036, 16.9149) projected
  line L65 (-14.8549, 16.5709) -> (-14.8856, 16.7658) projected
  line L66 (-14.8166, 16.381) -> (-14.8549, 16.5709) projected
  line L67 (-14.7703, 16.1965) -> (-14.8166, 16.381) projected
  line L68 (-14.7157, 16.0179) -> (-14.7703, 16.1965) projected
  line L69 (-14.6523, 15.8459) -> (-14.7157, 16.0179) projected
  line L70 (-14.5789, 15.6817) -> (-14.6523, 15.8459) projected
  line L71 (-14.4931, 15.5277) -> (-14.5789, 15.6817) projected
  line L72 (-14.446, 15.4541) -> (-14.4931, 15.5277) projected
  line L73 (-14.4047, 15.3757) -> (-14.446, 15.4541) projected
  line L74 (-14.3728, 15.2891) -> (-14.4047, 15.3757) projected
  line L75 (-14.3628, 15.2406) -> (-14.3728, 15.2891) projected
  line L76 (-14.3607, 15.1852) -> (-14.3628, 15.2406) projected
  line L77 (-14.4021, 15.0912) -> (-14.3607, 15.1852) projected
  line L78 (-15.0912, 14.4021) -> (-14.4021, 15.0912) projected
  line L79 (-15.1852, 14.3607) -> (-15.0912, 14.4021) projected
  line L80 (-15.2406, 14.3628) -> (-15.1852, 14.3607) projected
  line L81 (-15.2891, 14.3728) -> (-15.2406, 14.3628) projected
  line L82 (-15.3757, 14.4047) -> (-15.2891, 14.3728) projected
  line L83 (-15.4541, 14.446) -> (-15.3757, 14.4047) projected
  line L84 (-15.5277, 14.4931) -> (-15.4541, 14.446) projected
  line L85 (-15.6817, 14.5789) -> (-15.5277, 14.4931) projected
  line L86 (-15.8459, 14.6523) -> (-15.6817, 14.5789) projected
  line L87 (-16.0179, 14.7157) -> (-15.8459, 14.6523) projected
  line L88 (-16.1965, 14.7703) -> (-16.0179, 14.7157) projected
  line L89 (-16.381, 14.8166) -> (-16.1965, 14.7703) projected
  line L90 (-16.5709, 14.8549) -> (-16.381, 14.8166) projected
  line L91 (-16.7658, 14.8856) -> (-16.5709, 14.8549) projected
  line L92 (-16.9149, 14.9036) -> (-16.7658, 14.8856) projected
  line L93 (-17.5222, 13.9947) -> (-16.9149, 14.9036) projected
  line L94 (-17.4485, 13.8638) -> (-17.5222, 13.9947) projected
  line L95 (-17.3456, 13.6956) -> (-17.4485, 13.8638) projected
  line L96 (-17.2375, 13.5348) -> (-17.3456, 13.6956) projected
  line L97 (-17.1241, 13.382) -> (-17.2375, 13.5348) projected
  line L98 (-17.0053, 13.2378) -> (-17.1241, 13.382) projected
  line L99 (-16.8809, 13.1032) -> (-17.0053, 13.2378) projected
  line L100 (-16.7503, 12.9796) -> (-16.8809, 13.1032) projected
  line L101 (-16.6121, 12.8702) -> (-16.7503, 12.9796) projected
  line L102 (-16.5404, 12.8203) -> (-16.6121, 12.8702) projected
  line L103 (-16.4722, 12.7636) -> (-16.5404, 12.8203) projected
  line L104 (-16.4097, 12.6958) -> (-16.4722, 12.7636) projected
  line L105 (-16.3819, 12.6548) -> (-16.4097, 12.6958) projected
  line L106 (-16.3587, 12.6044) -> (-16.3819, 12.6548) projected
  line L107 (-16.3609, 12.5018) -> (-16.3587, 12.6044) projected
  line L108 (-16.7339, 11.6014) -> (-16.3609, 12.5018) projected
  line L109 (-16.8049, 11.5272) -> (-16.7339, 11.6014) projected
  line L110 (-16.8569, 11.5079) -> (-16.8049, 11.5272) projected
  line L111 (-16.9055, 11.4986) -> (-16.8569, 11.5079) projected
  line L112 (-16.9977, 11.4949) -> (-16.9055, 11.4986) projected
  line L113 (-17.086, 11.5031) -> (-16.9977, 11.4949) projected
  line L114 (-17.172, 11.5185) -> (-17.086, 11.5031) projected
  line L115 (-17.3471, 11.5388) -> (-17.172, 11.5185) projected
  line L116 (-17.5269, 11.5437) -> (-17.3471, 11.5388) projected
  line L117 (-17.71, 11.5365) -> (-17.5269, 11.5437) projected
  line L118 (-17.896, 11.5186) -> (-17.71, 11.5365) projected
  line L119 (-18.0842, 11.4907) -> (-17.896, 11.5186) projected
  line L120 (-18.2743, 11.4535) -> (-18.0842, 11.4907) projected
  line L121 (-18.466, 11.4073) -> (-18.2743, 11.4535) projected
  line L122 (-18.6107, 11.3669) -> (-18.466, 11.4073) projected
  line L123 (-18.824, 10.2947) -> (-18.6107, 11.3669) projected
  line L124 (-18.7058, 10.202) -> (-18.824, 10.2947) projected
  line L125 (-18.5463, 10.0859) -> (-18.7058, 10.202) projected
  line L126 (-18.3849, 9.9788) -> (-18.5463, 10.0859) projected
  line L127 (-18.2217, 9.881) -> (-18.3849, 9.9788) projected
  line L128 (-18.0568, 9.7933) -> (-18.2217, 9.881) projected
  line L129 (-17.8903, 9.7165) -> (-18.0568, 9.7933) projected
  line L130 (-17.7224, 9.6523) -> (-17.8903, 9.7165) projected
  line L131 (-17.5528, 9.604) -> (-17.7224, 9.6523) projected
  line L132 (-17.4675, 9.5854) -> (-17.5528, 9.604) projected
  line L133 (-17.3828, 9.5591) -> (-17.4675, 9.5854) projected
  line L134 (-17.299, 9.5204) -> (-17.3828, 9.5591) projected
  line L135 (-17.2577, 9.4932) -> (-17.299, 9.5204) projected
  line L136 (-17.217, 9.4555) -> (-17.2577, 9.4932) projected
  line L137 (-17.1798, 9.3598) -> (-17.217, 9.4555) projected
  line L138 (-17.1798, 8.3852) -> (-17.1798, 9.3598) projected
  line L139 (-17.217, 8.2895) -> (-17.1798, 8.3852) projected
  line L140 (-17.2577, 8.2518) -> (-17.217, 8.2895) projected
  line L141 (-17.299, 8.2246) -> (-17.2577, 8.2518) projected
  line L142 (-17.3828, 8.1859) -> (-17.299, 8.2246) projected
  line L143 (-17.4675, 8.1596) -> (-17.3828, 8.1859) projected
  line L144 (-17.5528, 8.141) -> (-17.4675, 8.1596) projected
  line L145 (-17.7224, 8.0927) -> (-17.5528, 8.141) projected
  line L146 (-17.8903, 8.0285) -> (-17.7224, 8.0927) projected
  line L147 (-18.0568, 7.9518) -> (-17.8903, 8.0285) projected
  line L148 (-18.2217, 7.864) -> (-18.0568, 7.9518) projected
  line L149 (-18.3849, 7.7662) -> (-18.2217, 7.864) projected
  line L150 (-18.5463, 7.6591) -> (-18.3849, 7.7662) projected
  line L151 (-18.7058, 7.543) -> (-18.5463, 7.6591) projected
  line L152 (-18.824, 7.4504) -> (-18.7058, 7.543) projected
  line L153 (-18.6107, 6.3782) -> (-18.824, 7.4504) projected
  line L154 (-18.466, 6.3378) -> (-18.6107, 6.3782) projected
  line L155 (-18.2743, 6.2915) -> (-18.466, 6.3378) projected
  line L156 (-18.0842, 6.2543) -> (-18.2743, 6.2915) projected
  line L157 (-17.896, 6.2264) -> (-18.0842, 6.2543) projected
  line L158 (-17.71, 6.2085) -> (-17.896, 6.2264) projected
  line L159 (-17.5269, 6.2013) -> (-17.71, 6.2085) projected
  line L160 (-17.3471, 6.2063) -> (-17.5269, 6.2013) projected
  line L161 (-17.172, 6.2266) -> (-17.3471, 6.2063) projected
  line L162 (-17.086, 6.242) -> (-17.172, 6.2266) projected
  line L163 (-16.9977, 6.2501) -> (-17.086, 6.242) projected
  line L164 (-16.9055, 6.2464) -> (-16.9977, 6.2501) projected
  line L165 (-16.8569, 6.2371) -> (-16.9055, 6.2464) projected
  line L166 (-16.8049, 6.2178) -> (-16.8569, 6.2371) projected
  line L167 (-16.7339, 6.1437) -> (-16.8049, 6.2178) projected
  line L168 (-16.3609, 5.2433) -> (-16.7339, 6.1437) projected
  line L169 (-16.3587, 5.1406) -> (-16.3609, 5.2433) projected
  line L170 (-16.3819, 5.0902) -> (-16.3587, 5.1406) projected
  line L171 (-16.4097, 5.0493) -> (-16.3819, 5.0902) projected
  line L172 (-16.4722, 4.9814) -> (-16.4097, 5.0493) projected
  line L173 (-16.5404, 4.9247) -> (-16.4722, 4.9814) projected
  line L174 (-16.6121, 4.8749) -> (-16.5404, 4.9247) projected
  line L175 (-16.7503, 4.7654) -> (-16.6121, 4.8749) projected
  line L176 (-16.8809, 4.6418) -> (-16.7503, 4.7654) projected
  line L177 (-17.0053, 4.5072) -> (-16.8809, 4.6418) projected
  line L178 (-17.1241, 4.363) -> (-17.0053, 4.5072) projected
  line L179 (-17.2375, 4.2102) -> (-17.1241, 4.363) projected
  line L180 (-17.3456, 4.0495) -> (-17.2375, 4.2102) projected
  line L181 (-17.4485, 3.8812) -> (-17.3456, 4.0495) projected
  line L182 (-17.5222, 3.7504) -> (-17.4485, 3.8812) projected
  line L183 (-16.9149, 2.8414) -> (-17.5222, 3.7504) projected
  line L184 (-16.7658, 2.8594) -> (-16.9149, 2.8414) projected
  line L185 (-16.5709, 2.8901) -> (-16.7658, 2.8594) projected
  line L186 (-16.381, 2.9285) -> (-16.5709, 2.8901) projected
  line L187 (-16.1965, 2.9747) -> (-16.381, 2.9285) projected
  line L188 (-16.0179, 3.0293) -> (-16.1965, 2.9747) projected
  line L189 (-15.8459, 3.0927) -> (-16.0179, 3.0293) projected
  line L190 (-15.6817, 3.1661) -> (-15.8459, 3.0927) projected
  line L191 (-15.5277, 3.2519) -> (-15.6817, 3.1661) projected
  line L192 (-15.4541, 3.299) -> (-15.5277, 3.2519) projected
  line L193 (-15.3757, 3.3403) -> (-15.4541, 3.299) projected
  line L194 (-15.2891, 3.3722) -> (-15.3757, 3.3403) projected
  line L195 (-15.2406, 3.3822) -> (-15.2891, 3.3722) projected
  line L196 (-15.1852, 3.3843) -> (-15.2406, 3.3822) projected
  line L197 (-15.0912, 3.3429) -> (-15.1852, 3.3843) projected
  line L198 (-14.4021, 2.6538) -> (-15.0912, 3.3429) projected
  line L199 (-14.3607, 2.5599) -> (-14.4021, 2.6538) projected
  line L200 (-14.3628, 2.5044) -> (-14.3607, 2.5599) projected
  line L201 (-14.3728, 2.4559) -> (-14.3628, 2.5044) projected
  line L202 (-14.4047, 2.3693) -> (-14.3728, 2.4559) projected
  line L203 (-14.446, 2.2909) -> (-14.4047, 2.3693) projected
  line L204 (-14.4931, 2.2174) -> (-14.446, 2.2909) projected
  line L205 (-14.5789, 2.0633) -> (-14.4931, 2.2174) projected
  line L206 (-14.6523, 1.8991) -> (-14.5789, 2.0633) projected
  line L207 (-14.7157, 1.7272) -> (-14.6523, 1.8991) projected
  line L208 (-14.7703, 1.5485) -> (-14.7157, 1.7272) projected
  line L209 (-14.8166, 1.364) -> (-14.7703, 1.5485) projected
  line L210 (-14.8549, 1.1741) -> (-14.8166, 1.364) projected
  line L211 (-14.8856, 0.9793) -> (-14.8549, 1.1741) projected
  line L212 (-14.9036, 0.8302) -> (-14.8856, 0.9793) projected
  line L213 (-13.9947, 0.2228) -> (-14.9036, 0.8302) projected
  line L214 (-13.8638, 0.2965) -> (-13.9947, 0.2228) projected
  line L215 (-13.6956, 0.3994) -> (-13.8638, 0.2965) projected
  line L216 (-13.5348, 0.5075) -> (-13.6956, 0.3994) projected
  line L217 (-13.382, 0.6209) -> (-13.5348, 0.5075) projected
  line L218 (-13.2378, 0.7397) -> (-13.382, 0.6209) projected
  line L219 (-13.1032, 0.8641) -> (-13.2378, 0.7397) projected
  line L220 (-12.9796, 0.9947) -> (-13.1032, 0.8641) projected
  line L221 (-12.8702, 1.1329) -> (-12.9796, 0.9947) projected
  line L222 (-12.8203, 1.2046) -> (-12.8702, 1.1329) projected
  line L223 (-12.7636, 1.2728) -> (-12.8203, 1.2046) projected
  line L224 (-12.6958, 1.3354) -> (-12.7636, 1.2728) projected
  line L225 (-12.6548, 1.3631) -> (-12.6958, 1.3354) projected
  line L226 (-12.6044, 1.3863) -> (-12.6548, 1.3631) projected
  line L227 (-12.5018, 1.3841) -> (-12.6044, 1.3863) projected
  line L228 (-11.6014, 1.0111) -> (-12.5018, 1.3841) projected
  line L229 (-11.5272, 0.9401) -> (-11.6014, 1.0111) projected
  line L230 (-11.5079, 0.8881) -> (-11.5272, 0.9401) projected
  line L231 (-11.4986, 0.8395) -> (-11.5079, 0.8881) projected
  line L232 (-11.4949, 0.7473) -> (-11.4986, 0.8395) projected
  line L233 (-11.5031, 0.659) -> (-11.4949, 0.7473) projected
  line L234 (-11.5185, 0.573) -> (-11.5031, 0.659) projected
  line L235 (-11.5388, 0.3979) -> (-11.5185, 0.573) projected
  line L236 (-11.5437, 0.2181) -> (-11.5388, 0.3979) projected
  line L237 (-11.5365, 0.035) -> (-11.5437, 0.2181) projected
  line L238 (-11.5186, -0.151) -> (-11.5365, 0.035) projected
  line L239 (-11.4907, -0.3392) -> (-11.5186, -0.151) projected
  line L240 (-11.4535, -0.5293) -> (-11.4907, -0.3392) projected
  line L241 (-11.4073, -0.721) -> (-11.4535, -0.5293) projected
  line L242 (-11.3669, -0.8657) -> (-11.4073, -0.721) projected
  line L243 (-10.2947, -1.0789) -> (-11.3669, -0.8657) projected
  line L244 (-10.202, -0.9608) -> (-10.2947, -1.0789) projected
  line L245 (-10.0859, -0.8013) -> (-10.202, -0.9608) projected
  line L246 (-9.9788, -0.6399) -> (-10.0859, -0.8013) projected
  line L247 (-9.881, -0.4767) -> (-9.9788, -0.6399) projected
  line L248 (-9.7933, -0.3118) -> (-9.881, -0.4767) projected
  line L249 (-9.7165, -0.1453) -> (-9.7933, -0.3118) projected
  line L250 (-9.6523, 0.0227) -> (-9.7165, -0.1453) projected
  line L251 (-9.604, 0.1922) -> (-9.6523, 0.0227) projected
  line L252 (-9.5854, 0.2775) -> (-9.604, 0.1922) projected
  line L253 (-9.5591, 0.3622) -> (-9.5854, 0.2775) projected
  line L254 (-9.5204, 0.446) -> (-9.5591, 0.3622) projected
  line L255 (-9.4932, 0.4873) -> (-9.5204, 0.446) projected
  line L256 (-9.4555, 0.528) -> (-9.4932, 0.4873) projected
  line L257 (-9.3598, 0.5652) -> (-9.4555, 0.528) projected
  line L258 (-8.3852, 0.5652) -> (-9.3598, 0.5652) projected
  line L259 (-8.2895, 0.528) -> (-8.3852, 0.5652) projected
  line L260 (-8.2518, 0.4873) -> (-8.2895, 0.528) projected
  line L261 (-8.2246, 0.446) -> (-8.2518, 0.4873) projected
  line L262 (-8.1859, 0.3622) -> (-8.2246, 0.446) projected
  line L263 (-8.1596, 0.2775) -> (-8.1859, 0.3622) projected
  line L264 (-8.141, 0.1922) -> (-8.1596, 0.2775) projected
  line L265 (-8.0927, 0.0227) -> (-8.141, 0.1922) projected
  line L266 (-8.0285, -0.1453) -> (-8.0927, 0.0227) projected
  line L267 (-7.9518, -0.3118) -> (-8.0285, -0.1453) projected
  line L268 (-7.864, -0.4767) -> (-7.9518, -0.3118) projected
  line L269 (-7.7662, -0.6399) -> (-7.864, -0.4767) projected
  line L270 (-7.6591, -0.8013) -> (-7.7662, -0.6399) projected
  line L271 (-7.543, -0.9608) -> (-7.6591, -0.8013) projected
  line L272 (-7.4504, -1.0789) -> (-7.543, -0.9608) projected
  line L273 (-6.3782, -0.8657) -> (-7.4504, -1.0789) projected
  line L274 (-6.3378, -0.721) -> (-6.3782, -0.8657) projected
  line L275 (-6.2915, -0.5293) -> (-6.3378, -0.721) projected
  line L276 (-6.2543, -0.3392) -> (-6.2915, -0.5293) projected
  line L277 (-6.2264, -0.151) -> (-6.2543, -0.3392) projected
  line L278 (-6.2085, 0.035) -> (-6.2264, -0.151) projected
  line L279 (-6.2013, 0.2181) -> (-6.2085, 0.035) projected
  line L280 (-6.2063, 0.3979) -> (-6.2013, 0.2181) projected
  line L281 (-6.2266, 0.573) -> (-6.2063, 0.3979) projected
  line L282 (-6.242, 0.659) -> (-6.2266, 0.573) projected
  line L283 (-6.2501, 0.7473) -> (-6.242, 0.659) projected
  line L284 (-6.2464, 0.8395) -> (-6.2501, 0.7473) projected
  line L285 (-6.2371, 0.8881) -> (-6.2464, 0.8395) projected
  line L286 (-6.2178, 0.9401) -> (-6.2371, 0.8881) projected
  line L287 (-6.1437, 1.0111) -> (-6.2178, 0.9401) projected
  line L288 (-5.2433, 1.3841) -> (-6.1437, 1.0111) projected
  line L289 (-5.1406, 1.3863) -> (-5.2433, 1.3841) projected
  line L290 (-5.0902, 1.3631) -> (-5.1406, 1.3863) projected
  line L291 (-5.0493, 1.3354) -> (-5.0902, 1.3631) projected
  line L292 (-4.9814, 1.2728) -> (-5.0493, 1.3354) projected
  line L293 (-4.9247, 1.2046) -> (-4.9814, 1.2728) projected
  line L294 (-4.8749, 1.1329) -> (-4.9247, 1.2046) projected
  line L295 (-4.7654, 0.9947) -> (-4.8749, 1.1329) projected
  line L296 (-4.6418, 0.8641) -> (-4.7654, 0.9947) projected
  line L297 (-4.5072, 0.7397) -> (-4.6418, 0.8641) projected
  line L298 (-4.363, 0.6209) -> (-4.5072, 0.7397) projected
  line L299 (-4.2102, 0.5075) -> (-4.363, 0.6209) projected
  line L300 (-4.0495, 0.3994) -> (-4.2102, 0.5075) projected
  line L301 (-3.8812, 0.2965) -> (-4.0495, 0.3994) projected
  line L302 (-3.7504, 0.2228) -> (-3.8812, 0.2965) projected
  line L303 (-2.8414, 0.8302) -> (-3.7504, 0.2228) projected
  line L304 (-2.8594, 0.9793) -> (-2.8414, 0.8302) projected
  line L305 (-2.8901, 1.1741) -> (-2.8594, 0.9793) projected
  line L306 (-2.9285, 1.364) -> (-2.8901, 1.1741) projected
  line L307 (-2.9747, 1.5485) -> (-2.9285, 1.364) projected
  line L308 (-3.0293, 1.7272) -> (-2.9747, 1.5485) projected
  line L309 (-3.0927, 1.8991) -> (-3.0293, 1.7272) projected
  line L310 (-3.1661, 2.0633) -> (-3.0927, 1.8991) projected
  line L311 (-3.2519, 2.2174) -> (-3.1661, 2.0633) projected
  line L312 (-3.299, 2.2909) -> (-3.2519, 2.2174) projected
  line L313 (-3.3403, 2.3693) -> (-3.299, 2.2909) projected
  line L314 (-3.3722, 2.4559) -> (-3.3403, 2.3693) projected
  line L315 (-3.3822, 2.5044) -> (-3.3722, 2.4559) projected
  line L316 (-3.3843, 2.5599) -> (-3.3822, 2.5044) projected
  line L317 (-3.3429, 2.6538) -> (-3.3843, 2.5599) projected
  line L318 (-2.6538, 3.3429) -> (-3.3429, 2.6538) projected
  line L319 (-2.5599, 3.3843) -> (-2.6538, 3.3429) projected
  line L320 (-2.5044, 3.3822) -> (-2.5599, 3.3843) projected
  line L321 (-2.4559, 3.3722) -> (-2.5044, 3.3822) projected
  line L322 (-2.3693, 3.3403) -> (-2.4559, 3.3722) projected
  line L323 (-2.2909, 3.299) -> (-2.3693, 3.3403) projected
  line L324 (-2.2174, 3.2519) -> (-2.2909, 3.299) projected
  line L325 (-2.0633, 3.1661) -> (-2.2174, 3.2519) projected
  line L326 (-1.8991, 3.0927) -> (-2.0633, 3.1661) projected
  line L327 (-1.7272, 3.0293) -> (-1.8991, 3.0927) projected
  line L328 (-1.5485, 2.9747) -> (-1.7272, 3.0293) projected
  line L329 (-1.364, 2.9285) -> (-1.5485, 2.9747) projected
  line L330 (-1.1741, 2.8901) -> (-1.364, 2.9285) projected
  line L331 (-0.9793, 2.8594) -> (-1.1741, 2.8901) projected
  line L332 (-0.8302, 2.8414) -> (-0.9793, 2.8594) projected
  line L333 (-0.2228, 3.7504) -> (-0.8302, 2.8414) projected
  line L334 (-0.2965, 3.8812) -> (-0.2228, 3.7504) projected
  line L335 (-0.3994, 4.0495) -> (-0.2965, 3.8812) projected